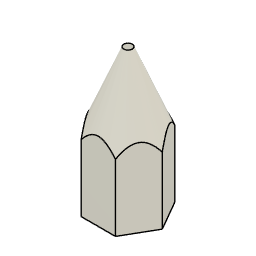
schibler-mathilde-1_carandache (Autodesk Fusion 360 design; units mm, degrees)
Autodesk Fusion 360 part; units mm, degrees
sketch "Esquisse1" plane through (0, 0, 0) normal (0, 1, 0) x (1, 0, 0)
  line L0 (11.547, -20) -> (23.094, 0)
  line L1 (23.094, 0) -> (11.547, 20)
  line L2 (11.547, 20) -> (-11.547, 20)
  line L3 (-11.547, 20) -> (-23.094, 0)
  line L4 (-23.094, 0) -> (-11.547, -20)
  line L5 (-11.547, -20) -> (11.547, -20)
  dimension "d1" = 20
  measures "d1" distance of origin L5
extrude "Extrusion1" add sketch "Esquisse1" along normal blind 95
sketch "Esquisse3" plane through (0, 0, 0) normal (0, 0, 1) x (1, 0, 0)
  line L0 (11.547, 95) -> (-11.547, 95)
  line L1 (-2.8927, 95) -> (-23.094, 45)
  line L2 (-23.094, 45) -> (-23.094, 95)
  line L3 (-23.094, 95) -> (-2.8927, 95)
  line L4 (-23.094, 0) -> (-23.094, 95)
  point P0 (0, 95)
  dimension "d8" = 50
  dimension "d9" = 22
  constraint coincident L0 L1.start
  constraint perpendicular L0 L2
  constraint horizontal L3
  constraint coincident L1.end L4
  measures "d8" distance of L1.end L2.end
  measures "d9" angle of L1 L2
revolve "Révolution1" cut sketch "Esquisse3" angle 360 about axis through (0, 1.75, 0) along (0, 1, 0)
extrude "Extrusion2" cut 1 faces at (0.2146, 95, -0.8551) along direction (0, -1, 0) blind 130
hole "Perçage1" at (0, 0, 0) direction (0, 1, 0) diameter 30 depth 40 tip angle 180
